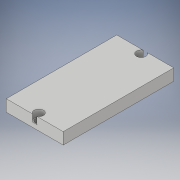
# Autodesk Inventor part: Bottom
Saved by Autodesk Inventor 2019 (Build 230136000, 136)
## iProperties
Created: 2020-02-01
Part Number: Bottom
Material: Generic
Document SubType Name: Modeling
Designer: alb16148
Density: 1 g/cm^3
Appearance: Default
Author: alb16148
Autodesk Inventor part; units mm, degrees
ref_plane "YZ Plane" through (0, 0, 0) normal (1, 0, 0) x (0, 1, 0)
ref_plane "XZ Plane" through (0, 0, 0) normal (0, 1, 0) x (-1, 0, 0)
ref_plane "XY Plane" through (0, 0, 0) normal (0, 0, 1) x (1, 0, 0)
sketch "Sketch1" plane through (0, 0, 0) normal (0, 1, 0) x (-1, 0, 0)
  line L0 (12.25, 23.75) -> (-12.25, 23.75)
  line L1 (-12.25, 23.75) -> (-12.25, -23.75)
  line L2 (-12.25, -23.75) -> (12.25, -23.75)
  line L3 (12.25, -23.75) -> (12.25, 23.75)
  point P0 (0, 0)
  dimension "d0" = 12.25
  dimension "d1" = 12.25
  dimension "d2" = 23.75
  dimension "d3" = 23.75
  constraints: 8 end point, 2 parallel, 1 horizontal, 1 perpendicular
  measures "d0" distance from line of L3 point (0, 0)
  measures "d1" distance from line of L1 point (0, 0)
  measures "d2" distance from line of L0 point (0, 0)
  measures "d3" distance from line of L2 point (0, 0)
extrude "Extrusion1" add sketch "Sketch1" along normal blind 5
sketch "Sketch2" plane through (0, 5, 0) normal (0, 1, 0) x (1, 0, 0)
  circle A0 centre (0, -22) radius 1.5
  circle A1 centre (0, 22) radius 1.5
  point P0 (0, 0)
  dimension "d6" = 3
  dimension "d7" = 3
  dimension "d8" = 22
  dimension "d9" = 22
  dimension "d10" = 0
  dimension "d11" = 0
  constraints: 2 centre point
  measures "d6" diameter of A0
  measures "d7" diameter of A1
  measures "d8" distance of A0.centre point (0, 0)
  measures "d9" distance of point (0, 0) A1.centre
  measures "d10" horizontal distance of point (0, 0) A0.centre
  measures "d11" horizontal distance of point (0, 0) A1.centre
extrude "Extrusion2" cut sketch "Sketch2" against normal up to surface (5 mm away)
sketch "Sketch4" plane through (0, 5, 0) normal (0, 1, 0) x (1, 0, 0)
  circle A0 centre (0, -22) radius 1.5 projected
  circle A1 centre (0, 22) radius 1.5 projected
  line L0 (-12.25, -23.75) -> (12.25, -23.75) projected
  line L1 (12.25, -23.75) -> (12.25, 23.75) projected
  line L2 (12.25, 23.75) -> (-12.25, 23.75) projected
  line L3 (-12.25, 23.75) -> (-12.25, -23.75) projected
  circle A2 centre (0, -22) radius 2
  circle A3 centre (0, 22) radius 2
  point P0 (0, 0)
  dimension "d14" = 4
  dimension "d15" = 4
  constraints: 2 centre point, 2 coincident
  measures "d14" diameter of A2
  measures "d15" diameter of A3
extrude "Extrusion3" cut sketch "Sketch4" against normal blind 3 contours A2 L0 | L0 A2 | A3 L2 | L2 A3
sketch "Sketch5" plane through (0, 0, 0) normal (0, -1, 0) x (1, 0, 0)
  line L0 (-12.25, -23.75) -> (-12.25, 23.75) projected
  line L1 (-12.25, 23.75) -> (12.25, 23.75) projected
  line L2 (12.25, -23.75) -> (-12.25, -23.75) projected
  line L3 (10.15, 19.65) -> (-10.15, 19.65)
  line L4 (-10.15, 19.65) -> (-10.15, -19.65)
  line L5 (-10.15, -19.65) -> (10.15, -19.65)
  line L6 (10.15, -19.65) -> (10.15, 19.65)
  line L7 (12.25, 23.75) -> (12.25, -23.75) projected
  point P0 (0, 0)
  dimension "d20" = 4.1
  dimension "d21" = 4.1
  dimension "d22" = 2.1
  dimension "d23" = 2.1
  constraints: 8 end point, 2 parallel, 1 horizontal, 1 perpendicular
  measures "d20" distance between parallel lines of L1 L3
  measures "d21" distance between parallel lines of L5 L2
  measures "d22" distance between parallel lines of L7 L6
  measures "d23" distance between parallel lines of L4 L0
extrude "Extrusion4" cut sketch "Sketch5" against normal blind 2 contours L6 L5 L4 L3
equation "\"d1\" = d0"
equation "\"d3\" = d2"
equation "\"d21\" = d20"
equation "\"d23\" = d22"
body "Solid1"
